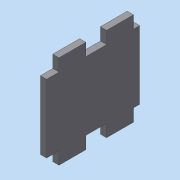
# Autodesk Inventor part: X-Anchor_Inner
Saved by Autodesk Inventor 2016 SP1 (Build 200210100, 210)
## iProperties
Created: 2016-03-02
Part Number: X-Anchor_Inner
Material: Generic
Document SubType Name: Modeling
Designer: Mohamed A.
Density: 1 g/cm^3
Appearance: Default
Author: Mohamed A.
Autodesk Inventor part; units mm, degrees
ref_plane "YZ Plane" through (0, 0, 0) normal (1, 0, 0) x (0, 1, 0)
ref_plane "XZ Plane" through (0, 0, 0) normal (0, 1, 0) x (-1, 0, 0)
ref_plane "XY Plane" through (0, 0, 0) normal (0, 0, 1) x (1, 0, 0)
sketch "Sketch2" plane through (0, 0, 0) normal (1, 0, 0) x (0, 1, 0)
  line L0 (22.5, 16.5) -> (19.5, 16.5)
  line L1 (-22.5, 16.5) -> (-22.5, -16.5)
  line L2 (-22.5, -16.5) -> (-16.5, -16.5)
  line L3 (22.5, -16.5) -> (22.5, 16.5)
  line L4 (22.5, 16.5) -> (-22.5, -16.5) construction
  line L5 (-22.5, 16.5) -> (22.5, -16.5) construction
  line L6 (19.5, -16.5) -> (19.5, -22.5)
  line L7 (19.5, -22.5) -> (6.5, -22.5)
  line L8 (6.5, -22.5) -> (6.5, -16.5)
  line L9 (-3.5, -16.5) -> (-3.5, -22.5)
  line L10 (-3.5, -22.5) -> (-16.5, -22.5)
  line L11 (-16.5, -22.5) -> (-16.5, -16.5)
  line L12 (-35.1, 0) -> (32.1, 0) construction
  line L13 (0, -31.5) -> (0, 31.5) construction
  line L14 (19.5, 16.5) -> (19.5, 22.5)
  line L15 (19.5, 22.5) -> (6.5, 22.5)
  line L16 (6.5, 22.5) -> (6.5, 16.5)
  line L17 (-3.5, 16.5) -> (-3.5, 22.5)
  line L18 (-3.5, 22.5) -> (-16.5, 22.5)
  line L19 (-16.5, 22.5) -> (-16.5, 16.5)
  line L20 (19.5, -16.5) -> (22.5, -16.5)
  line L21 (6.5, -16.5) -> (19.5, -16.5)
  line L22 (-3.5, -16.5) -> (6.5, -16.5)
  line L23 (-16.5, -16.5) -> (-3.5, -16.5)
  line L24 (-16.5, 16.5) -> (-22.5, 16.5)
  line L25 (-3.5, 16.5) -> (-16.5, 16.5)
  line L26 (6.5, 16.5) -> (-3.5, 16.5)
  line L27 (19.5, 16.5) -> (6.5, 16.5)
  line L28 (-22.5, -7.5) -> (-25.5, -7.5)
  line L29 (-25.5, -7.5) -> (-25.5, 7.5)
  line L30 (-25.5, 7.5) -> (-22.5, 7.5)
  point P0 (0, 0)
  dimension "d0" = 45
  dimension "d1" = 33
  dimension "d4" = 6
  dimension "d5" = 3
  dimension "d6" = 13
  dimension "d7" = 13
  dimension "d8" = 10
  dimension "d9" = 3
  dimension "d10" = 9
  constraints: 58 end point, 26 parallel, 19 perpendicular, 8 symmetric about line, 6 horizontal, 2 midpoint, 2 point on line, 2 vertical, 1 collinear, 1 other
  measures "d0" distance of L3.start L1.end
  measures "d1" distance of L1.end L1.start
  measures "d4" distance of L6.start L6.end
  measures "d5" distance between parallel lines of L6 L3
  measures "d6" distance between parallel lines of L8 L6
  measures "d7" distance of L9.end L10.end
  measures "d8" distance between parallel lines of L9 L8
  measures "d9" distance of L28.start L28.end
  measures "d10" distance between parallel lines of L28 L2
extrude "Extrusion1" add sketch "Sketch2" along normal blind 3
body "Solid1"
